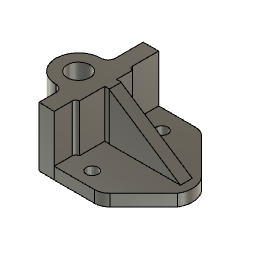
A3 (Autodesk Fusion 360 design; units mm, degrees)
Autodesk Fusion 360 part; units mm, degrees
sketch "Sketch1" plane through (0, 0, 0) normal (0, 0, 1) x (1, 0, 0)
  line L0 (16, -42.0976) -> (-21.8982, -42.0976)
  line L1 (-21.8982, 45.9024) -> (8.8992, 45.9024)
  circle A0 centre (-2.4953, 29.3056) radius 5
  circle A1 centre (-2.5166, -29.3521) radius 5
  line L2 (49.7533, -9.8697) -> (21.333, -38.29)
  line L3 (0, 0) -> (-2.2254, 0) construction
  line L4 (48.2962, 11.8902) -> (18.0915, 42.0948)
  line L5 (0, 0) -> (-2.144, 0) construction
  arc A2 (43.3404, -16.2826) -> (45.4196, 14.7668) centre (33.5001, -0.0293) ccw
  line L6 (-0.3569, 24.7859) -> (-0.3438, 23.7609) construction
  line L7 (0.266, -23.8067) -> (0.284, -25.21) construction
  arc A3 (-1.0393, 24.5222) -> (-0.3438, 23.7609) centre (8.8992, 32.9024) ccw
  arc A4 (21.89, 33.3903) -> (-2.0318, 39.9391) centre (8.8992, 32.9024) ccw
  arc A5 (1.9684, -37.1924) -> (21.333, -38.29) centre (12.1406, -29.0976) ccw
  arc A6 (0.266, -23.8067) -> (-0.1748, -24.9344) centre (12.1406, -29.0976) ccw
  line L8 (-21.8982, 45.9024) -> (-20, 45.9024) construction
  line L9 (-21.8982, 45.9024) -> (-34.8982, 45.9024)
  line L10 (-34.8982, -41.7625) -> (-21.8982, -42.0976)
  line L11 (-21.8982, 45.9024) -> (-21.8982, 23.9024) construction
  line L12 (-18.8982, 7.4942) -> (-14.8982, 7.4942)
  line L13 (-14.8982, -2.5058) -> (-14.8982, 7.4942)
  line L14 (-14.8982, -2.5058) -> (-18.8982, -2.5058)
  circle A7 centre (-40.8982, -2.5503) radius 9.5
  line L15 (-41.2845, 16.4458) -> (-40.512, 16.4458) construction
  line L16 (-34.8982, 45.9024) -> (-34.8982, 22.4458)
  line L17 (-41.0282, -21.5498) -> (-40.7683, -21.5498) construction
  arc A8 (-40.512, 16.4458) -> (-40.7683, -21.5498) centre (-40.8982, -2.5503) ccw
  line L18 (-34.8982, -27.5498) -> (-34.8982, -41.7625)
  line L19 (-21.8982, -42.0976) -> (-21.8982, -26.7935)
  line L20 (-21.8982, 23.9024) -> (-21.8982, 45.9024)
  arc A9 (-21.8982, 23.9024) -> (-18.8982, 20.9024) centre (-18.8982, 23.9024) ccw
  arc A10 (-34.8982, -27.5498) -> (-40.8982, -21.5498) centre (-40.8982, -27.5498) ccw
  arc A11 (-41.0874, 16.4488) -> (-34.8982, 22.4458) centre (-40.8982, 22.4458) ccw
  arc A12 (-18.8982, -23.7935) -> (-21.8982, -26.7935) centre (-18.8982, -26.7935) ccw
  line L21 (-18.8982, 20.9024) -> (-18.8982, 7.4942)
  line L22 (-18.8982, -2.5058) -> (-18.8982, -23.7935)
  dimension "d2" = 88
  dimension "d3" = 10
  dimension "d4" = 10
  dimension "d5" = 50
  dimension "d8" = 19
  dimension "d9" = 45
  dimension "d10" = 45
  dimension "d11" = 13
  dimension "d12" = 13
  dimension "d13" = 13
  dimension "d17" = 4
  dimension "d18" = 10
  dimension "d19" = 3
  dimension "d20" = 3
  dimension "d22" = 19
  dimension "d23" = 19
  dimension "d24" = 6
  dimension "d25" = 6
  constraint horizontal L0
  constraint perpendicular L0 L19
  constraint parallel L0 L1
  constraint coincident A0 L6.start
  constraint coincident A1 L7.end
  constraint horizontal L3
  constraint horizontal L5
  constraint tangent L4 A3
  constraint tangent L1 A3
  constraint tangent L2 A5
  constraint tangent L0 A5
  constraint coincident L2.start A2
  constraint coincident L4.start A2
  constraint coincident L1.end A3
  constraint coincident L4 A2.end
  constraint coincident L2 A2.start
  constraint coincident A4.start A3
  constraint coincident A1 A6.end
  constraint coincident A0 A3.start
  constraint collinear L6 L7
  constraint concentric A3 A4
  constraint coincident L7.start A5
  constraint concentric A5 A6
  constraint coincident A4 L4.end
  constraint coincident L1 L8.end
  constraint perpendicular L9 L19
  constraint perpendicular L9 L16
  constraint perpendicular L12 L21
  constraint perpendicular L12 L13
  constraint coincident L14.end L21
  constraint perpendicular L14 L21
  constraint tangent L19 A12
  constraint tangent L11 A9
  constraint concentric A7 A8
  constraint coincident L15.start A8
  constraint perpendicular L15 L21
  constraint coincident L17.start A8
  constraint horizontal L17
  constraint tangent L15 A11
  constraint tangent L16 A11
  constraint tangent L17 A10
  constraint tangent L16 A10
  constraint collinear L19 L20
  constraint coincident L17 A10.end
  constraint coincident A8 A11.start
  constraint collinear L21 L22
  measures "d2" distance of L0.end L1.start
  measures "d3" diameter of A0
  measures "d4" diameter of A1
  measures "d5" distance of L6.start L7.end
  measures "d8" radius of A2
  measures "d9" angle of L2 L3
  measures "d10" angle of L4 L5
  measures "d11" radius of A3
  measures "d12" radius of A5
  measures "d13" distance of L1.start L9.end
  measures "d17" distance of L12.start L12.end
  measures "d18" distance of L12.end L13.start
  measures "d19" radius of A12
  measures "d20" radius of A9
  measures "d22" radius of A8
  measures "d23" diameter of A7
  measures "d24" radius of A11
  measures "d25" radius of A10
extrude "Extrude1" add sketch "Sketch1" along normal blind 10 contours L0 L1 L2 L4 A2 A4 A5 L12 L13 L14 L19 L20 A9 A12 L21 L22
extrude "Extrude2" add sketch "Sketch1" along normal blind 50 contours L9 L10 L12 L13 L14 L16 A8 L18 L19 L20 A9 A10 A11 A12 L21 L22
sketch "Sketch2" plane through (0, 0, 0) normal (0, 1, 0) x (1, 0, 0)
  line L0 (-14.9, -50, 2.2444) -> (-14.9, -10, 2.2444)
  line L1 (-14.9, -10, 2.2444) -> (45.1, -10, 2.2444)
  line L2 (45.1, -10, 2.2444) -> (-14.9, -50, 2.2444)
  dimension "d30" = 40
  dimension "d31" = 60
extrude "Extrude4" add sketch "Sketch2" along normal mid plane 10 contours L0 L1 L2 in plane through (0, 2.2444, 0) normal (0, 1, 0)
extrude "Extrude3" [suppressed]
